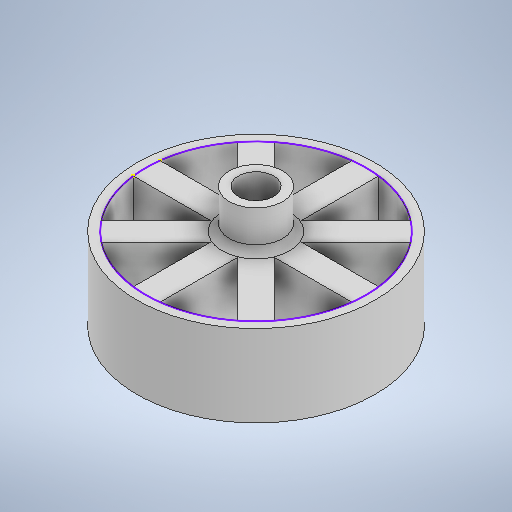
# Autodesk Inventor part: rueda de motol
Saved by Autodesk Inventor 2025.2 (Build 292293000, 293)
## iProperties
Created: 2025-04-22
Part Number: rueda de motol
Material: Generic
Document SubType Name: Modeling
Designer: maqmat
Density: 1 g/cm^3
Appearance: Default
Author: maqmat
Autodesk Inventor part; units mm, degrees
ref_plane "YZ Plane" through (0, 0, 0) normal (1, 0, 0) x (0, 1, 0)
ref_plane "XZ Plane" through (0, 0, 0) normal (0, 1, 0) x (-1, 0, 0)
ref_plane "XY Plane" through (0, 0, 0) normal (0, 0, 1) x (1, 0, 0)
sketch "Sketch1" plane through (0, 0, 0) normal (0, 1, 0) x (-1, 0, 0)
  circle A0 centre (0, 0) radius 31
  circle A1 centre (0, 0) radius 33.5
  dimension "d0" = 62
  dimension "d1" = 67
  constraints: 2 centre point, 2 coincident
  measures "d0" diameter of A0
  measures "d1" diameter of A1
extrude "Extrusion1" add sketch "Sketch1" along normal blind 23
sketch "Sketch3" plane through (0, 23, 0) normal (0, 1, 0) x (1, 0, 0)
  circle A0 centre (0, 0) radius 31
  constraints: 1 centre point, 1 coincident
hole "Hole1" at (0, 23, 0) direction (0, -1, 0) diameter 62 end through all
sketch "Sketch4" plane through (0, 23, 0) normal (0, 1, 0) x (1, 0, 0)
  circle A0 centre (0, 0) radius 9.4443
  constraints: 1 centre point, 1 coincident
hole "Hole2" at (0, 23, 0) direction (0, -1, 0) diameter 62 end through all
sketch "Sketch5" plane through (0, 0, 0) normal (0, -1, 0) x (1, 0, 0)
  circle A0 centre (0, 0) radius 5
  line L0 (-5, 2.5) -> (-30.9738, 2.5)
  line L1 (-5, -2.5) -> (-30.9738, -2.5)
  line L2 (-4.3301, 2.5) -> (-5, 2.5)
  line L3 (-5, -2.5) -> (-4.3301, -2.5)
  dimension "d46" = 10
  constraints: 8 end point, 3 horizontal, 2 point on circle, 1 centre point, 1 coincident, 1 collinear, 1 point on line
  measures "d46" diameter of A0
extrude "Extrusion3" add sketch "Sketch5" against normal blind 23
sketch "Sketch6" plane through (0, 23, 0) normal (0, 1, 0) x (1, 0, 0)
  circle A0 centre (0, 0) radius 7.5
  dimension "d49" = 15
  constraints: 1 centre point, 1 coincident
  measures "d49" diameter of A0
extrude "Extrusion4" add sketch "Sketch6" against normal blind 23
sketch "Sketch7" plane through (0, 23, 0) normal (0, 1, 0) x (1, 0, 0)
  circle A0 centre (0, 0) radius 5
  circle A1 centre (0, 0) radius 31 projected
  circle A2 centre (0, 0) radius 7.5
  dimension "d52" = 10
  constraints: 2 centre point, 2 coincident
  measures "d52" diameter of A0
extrude "Extrusion5" add sketch "Sketch7" along normal blind 11 contours A2
sketch "Sketch8" plane through (0, 0, 0) normal (0, -1, 0) x (1, 0, 0)
  circle A0 centre (0, 0) radius 7.5 projected
  line L0 (-6.4952, 3.75) -> (-30.7723, 3.75)
  circle A1 centre (0, 0) radius 31 projected
  line L1 (-6.4952, -3.75) -> (-30.7723, -3.75)
  line L2 (-1.9411, -7.2444) -> (-19.1077, -24.411)
  line L3 (-7.2444, -1.9411) -> (-24.411, -19.1077)
  line L4 (3.75, -6.4952) -> (3.75, -30.7723)
  line L5 (-3.75, -6.4952) -> (-3.75, -30.7723)
  line L6 (7.2444, -1.9411) -> (24.411, -19.1077)
  line L7 (1.9411, -7.2444) -> (19.1077, -24.411)
  line L8 (6.4952, 3.75) -> (30.7723, 3.75)
  line L9 (6.4952, -3.75) -> (30.7723, -3.75)
  line L10 (1.9411, 7.2444) -> (19.1077, 24.411)
  line L11 (7.2444, 1.9411) -> (24.411, 19.1077)
  line L12 (-3.75, 6.4952) -> (-3.75, 30.7723)
  line L13 (3.75, 6.4952) -> (3.75, 30.7723)
  line L14 (-7.2444, 1.9411) -> (-24.411, 19.1077)
  line L15 (-1.9411, 7.2444) -> (-19.1077, 24.411)
  point P0 (-9.0533, -3.75)
  point P1 (-3.75, -9.0533)
  point P2 (3.75, -9.0533)
  point P3 (9.0533, -3.75)
  point P4 (9.0533, 3.75)
  point P5 (3.75, 9.0533)
  point P6 (-3.75, 9.0533)
  point P7 (-9.0533, 3.75)
  dimension "d57" = 360
  constraints: 32 end point, 4 point on circle, 1 horizontal, 1 parallel, 49 other
extrude "Extrusion6" add sketch "Sketch8" against normal blind 23 contours A0 L11 L8 A1 L9 L6 | A0 L8 L11 | L6 L9 A0 | A0 L13 L10 A1 L11 L8 | L9 L6 A1 L7 L4 A0 | A0 L10 L13 | L4 L7 A0 | A0 L15 L12 A1 L13 L10 | L7 L4 A1 L5 L2 A0 | A0 L12 L15 | L2 L5 A0 | A0 L0 L14 A1 L15 L12 | L5 L2 A1 L3 L1 A0 | A0 L14 L0 | L1 L3 A0 | A0 L3 L1 A1 L0 L14
sketch "Sketch9" plane through (0, 23, 0) normal (0, 1, 0) x (1, 0, 0)
  circle A0 centre (0, 0) radius 7.5 projected
  circle A1 centre (0, 0) radius 7.5 projected
  circle A2 centre (0, 0) radius 7.5
  circle A3 centre (0, 0) radius 30.9985
  point P0 (-30.7723, 3.75)
  point P1 (-30.7723, -3.75)
  constraints: 2 centre point, 2 coincident
fillet "Fillet2" radius 2 1 edges at (-7.5, 23, 0)
body "Solid1"
